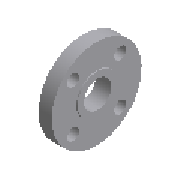
# Autodesk Inventor part: DIN EN 1092-2 Hubbed Slip-On Flange for Welding Type 12 - PN 63 Ductile Iron DN80
Saved by Autodesk Inventor 2024.2 (Build 282272000, 272)
## iProperties
Created: 2023-01-19
Part Number: DIN EN 1092-2 Hubbed Slip-On Flange for Welding Type 12 - PN 63 Ductile Iron DN80
Material: Iron, Ductile
Description: Flange
Document SubType Name: Modeling
Standard: DIN EN 1092-2
Designer: admin
Standards Organization: DIN
Language: en-US
Size Designation: DN80
Categories: <MemberInstance><Categories><Category DisplayName="Tube &amp; Pipe" InternalName="4347fa0f-2144-441d-94cd-e3e15c92b736" Mnemonic="TUBEANDPIPE"><CategoryParameter DisplayName="Number of Connections" InternalName="04e9c83a-9e20-4a98-a7e1-e8abe87a2846" Mnemonic="NUM_CONNECTIONS"/><CategoryParameter DisplayName="Angles" InternalName="0e0e4fa4-3bd3-4656-a22e-4e07c8c476f8" Mnemonic="ANGLES"><CategoryParameter DisplayName="Angle" InternalName="9188ad83-1b16-48b4-8b0a-76ce729dafa7" Mnemonic="ANGLE"/></CategoryParameter><CategoryParameter DisplayName="SKey" InternalName="3da84699-049a-4bc2-a65a-6696b77c242f" Mnemonic="SKEY"/><CategoryParameter DisplayName="ISOGEN Description" InternalName="7aa3ba45-b821-4467-8584-f9e6f15f2a7d" Mnemonic="ISOGENDESC"/><CategoryParameter DisplayName="ITEM-CODE" InternalName="99cc3b15-24d9-4d38-aac7-792cfbc57acf" Mnemonic="ITEMCODE"/><CategoryParameter DisplayName="NameOfComponent" InternalName="9c74ad13-48a1-45fe-b0f7-5447561f444a" Mnemonic="NAMEOFCOMPONENT"/><CategoryParameter DisplayName="InLineGroups" InternalName="d60be647-bc43-4c18-a13f-9fe4115f8e64" Mnemonic="INLINEGROUPS"/><Category DisplayName="Fittings" InternalName="ed6b26c4-72b8-4f31-9b63-f85ae8f932e4" Mnemonic="FITTINGS"><CategoryParameter DisplayName="Connections" InternalName="dbd721e8-e885-4eea-9011-b5acfd9f61de" Mnemonic="FIT_CONNECTIONS"><CategoryParameter DisplayName="Min Mating Pipe Size" InternalName="11f51b32-3e37-4310-abf7-f1318a1fd129" Mnemonic="MNMPS"/><CategoryParameter DisplayName="MaxEngagement" InternalName="34fdf028-8797-436e-ba07-ca3dee15bd9b" Mnemonic="MAXENGAGEMENT"/><CategoryParameter DisplayName="NominalSize" InternalName="3f94edc7-e459-48db-8f02-8eebf8cffccd" Mnemonic="NS"/><CategoryParameter DisplayName="DisplayName" InternalName="50f521dd-e050-43f7-9895-6b30ea7ed42e" Mnemonic="DISPLAYNAME"/><CategoryParameter DisplayName="Cut Mating Pipe" InternalName="53a63a6e-53d8-4ca9-8880-037731d1cceb" Mnemonic="CMP"/><CategoryParameter DisplayName="Gender Neutral" InternalName="628bd5f1-acad-44e2-9d91-af996ab74fc2" Mnemonic="NEUTRAL"/><CategoryParameter DisplayName="MinEngagement [% of MaxEngagement]" InternalName="7ec1bde5-73f0-45b1-98d8-365a6c67f8ad" Mnemonic="MINENGAGEMENT"/><CategoryParameter DisplayName="Fixed" InternalName="9142902a-6a8a-446d-9eb8-4b7ce7d245ef" Mnemonic="FIXED"/><CategoryParameter DisplayName="Female" InternalName="b366bcb5-a500-4bad-84bb-22f956216d69" Mnemonic="FEMALE"/><CategoryParameter DisplayName="FlipDirection" InternalName="d55dedc0-f14a-4283-86b4-a4eeb253c8aa" Mnemonic="FLIPDIRECTION"/><CategoryParameter DisplayName="ScheduleNumber" InternalName="d6161c62-eb59-4495-a086-874847c10866" Mnemonic="SN"/><CategoryParameter DisplayName="EndTreatment" InternalName="d7f11516-3374-45ca-b1c7-4b2d63244ae2" Mnemonic="ENDTREATMENT"/><CategoryParameter DisplayName="Max Mating Pipe Size" InternalName="e73ef66b-c04b-45ac-9b32-f712653e25ee" Mnemonic="MXMPS"/></CategoryParameter><CategoryParameter DisplayName="Connections" InternalName="dbd721e8-e885-4eea-9011-b5acfd9f61de" Mnemonic="FIT_CONNECTIONS"><CategoryParameter DisplayName="Min Mating Pipe Size" InternalName="11f51b32-3e37-4310-abf7-f1318a1fd129" Mnemonic="MNMPS"/><CategoryParameter DisplayName="MaxEngagement" InternalName="34fdf028-8797-436e-ba07-ca3dee15bd9b" Mnemonic="MAXENGAGEMENT"/><CategoryParameter DisplayName="NominalSize" InternalName="3f94edc7-e459-48db-8f02-8eebf8cffccd" Mnemonic="NS"/><CategoryParameter DisplayName="DisplayName" InternalName="50f521dd-e050-43f7-9895-6b30ea7ed42e" Mnemonic="DISPLAYNAME"/><CategoryParameter DisplayName="Cut Mating Pipe" InternalName="53a63a6e-53d8-4ca9-8880-037731d1cceb" Mnemonic="CMP"/><CategoryParameter DisplayName="Gender Neutral" InternalName="628bd5f1-acad-44e2-9d91-af996ab74fc2" Mnemonic="NEUTRAL"/><CategoryParameter DisplayName="MinEngagement [% of MaxEngagement]" InternalName="7ec1bde5-73f0-45b1-98d8-365a6c67f8ad" Mnemonic="MINENGAGEMENT"/><CategoryParameter DisplayName="Fixed" InternalName="9142902a-6a8a-446d-9eb8-4b7ce7d245ef" Mnemonic="FIXED"/><CategoryParameter DisplayName="Female" InternalName="b366bcb5-a500-4bad-84bb-22f956216d69" Mnemonic="FEMALE"/><CategoryParameter DisplayName="FlipDirection" InternalName="d55dedc0-f14a-4283-86b4-a4eeb253c8aa" Mnemonic="FLIPDIRECTION"/><CategoryParameter DisplayName="ScheduleNumber" InternalName="d6161c62-eb59-4495-a086-874847c10866" Mnemonic="SN"/><CategoryParameter DisplayName="EndTreatment" InternalName="d7f11516-3374-45ca-b1c7-4b2d63244ae2" Mnemonic="ENDTREATMENT"/><CategoryParameter DisplayName="Max Mating Pipe Size" InternalName="e73ef66b-c04b-45ac-9b32-f712653e25ee" Mnemonic="MXMPS"/></CategoryParameter><Category DisplayName="Flanges" InternalName="77d2c0aa-3125-426d-b447-5c3546f42b82" Mnemonic="Flange"/></Category></Category><Category DisplayName="DataType" InternalName="23b78d0f-2648-40c6-8793-ca6db495c9e8" Mnemonic="DATATYPE"><CategoryParameter DisplayName="DisplayName" InternalName="05415f3d-3907-474b-a020-eb9d644f4cf3" Mnemonic="DISPLAYNAME"/><CategoryParameter DisplayName="Standard" InternalName="0c0a119c-1e12-4c84-803f-101930972f5e" Mnemonic="STANDARD"/><CategoryParameter DisplayName="Description" InternalName="13903e3d-64b1-4950-80da-f627842ea37f" Mnemonic="DESCRIPTION"/><CategoryParameter DisplayName="Designation" InternalName="2675968c-4ce5-49e0-a4f5-552d29089031" Mnemonic="DESIGNATION"/><CategoryParameter DisplayName="Default Row" InternalName="2af9ec52-faaa-4026-b378-f9fa4afca842" Mnemonic="DEFAULTROW"/><CategoryParameter DisplayName="Folder Name" InternalName="3f06958e-8713-4116-9be7-ed6184ecc97b" Mnemonic="FOLDERNAME"/><CategoryParameter DisplayName="Revision Guid" InternalName="45a75005-10b1-4dfc-8d6d-dfe629f0b93c" Mnemonic="REVISIONGUID"/><CategoryParameter DisplayName="FileName" InternalName="8b46a4cc-9585-4fed-90c3-899f57e09a73" Mnemonic="FILENAME"/><CategoryParameter DisplayName="StdsOrg" InternalName="8f5914e1-4693-403f-8ab5-d37768198c9d" Mnemonic="STDSORG"/><CategoryParameter DisplayName="Family Version" InternalName="914462f6-6e19-4b14-ba84-155b9680b1d0" Mnemonic="FAMILYREVISION"/><CategoryParameter DisplayName="Standard Revision" InternalName="91d5a463-65c2-4fde-b823-3b7fea5e8e17" Mnemonic="STANDARDREVISION"/><CategoryParameter DisplayName="Member Revision" InternalName="a65d44b9-392f-4f4f-857b-e4b3d54996fe" Mnemonic="MEMBERREVISION"/><CategoryParameter DisplayName="ClipFormat" InternalName="bc51e27b-3422-4e78-93ef-cec197ddf230" Mnemonic="CLIPFORMAT"/><CategoryParameter DisplayName="Manufacturer" InternalName="cd6c7a72-a28a-4e50-99a9-2c7f4e13e5ad" Mnemonic="MANUFACTURER"/><CategoryParameter DisplayName="InternalName" InternalName="cf1d0246-76d9-4b4a-8305-fa0409afb5c1" Mnemonic="INTERNALNAME"/><CategoryParameter DisplayName="IsMetric" InternalName="e2385c5b-1ea4-4823-96a8-8de651266ec3" Mnemonic="ISMETRIC"/><Category DisplayName="Part" InternalName="c0e0b642-3bcb-4cc8-9e80-f96d35c4afa4" Mnemonic="PART"><CategoryParameter DisplayName="Part Number" InternalName="016b6077-bfbe-49bd-92c9-d8d59c39c941" Mnemonic="PARTNUMBER"/><CategoryParameter DisplayName="Stock Number" InternalName="4dba7c1c-e26c-444e-836c-b08b433409a8" Mnemonic="STOCKNUMBER"/><CategoryParameter DisplayName="Material Key" InternalName="5c9a8adb-dd2b-4535-b97f-0a94a95fe41f" Mnemonic="MATERIALKEY"/><CategoryParameter DisplayName="Material" InternalName="818a152a-d3c3-49ca-80ee-df7d91421b8e" Mnemonic="MATERIAL"/></Category></Category><Category DisplayName="LegacyMap" InternalName="dfeab48a-acc2-4514-a11c-1b8dc28c3d5f" Mnemonic="LEGACYMAP"><CategoryParameter DisplayName="CatalogID" InternalName="0da51c36-8fd3-4028-86cc-0c9c9e96136a" Mnemonic="CATALOGID"/><CategoryParameter DisplayName="FamilyID" InternalName="1c0b589c-8bbe-4e1e-80cf-07c0de42ac2a" Mnemonic="FAMILYID"/><CategoryParameter DisplayName="MemberID" InternalName="a368ea03-db8a-4d6e-962b-2aa46306b8f5" Mnemonic="MEMBERID"/></Category></Categories><FamilyTemplate Id="DIN EN 1092-2 Hubbed Slip-On Flange for Welding Type 12 - PN 63 Ductile Iron"><FamilyTemplateParameters><FamilyTemplateParameter ObjectType="kUserParameterObject" ValueType="xs:integer" Id="1" ObjectReferenceKey="NU"/><FamilyTemplateParameter ObjectType="kUserParameterObject" ValueType="xs:double" Id="2" ObjectReferenceKey="D"/><FamilyTemplateParameter ObjectType="kUserParameterObject" ValueType="xs:double" Id="3" ObjectReferenceKey="K1"/><FamilyTemplateParameter ObjectType="kUserParameterObject" ValueType="xs:double" Id="4" ObjectReferenceKey="L"/><FamilyTemplateParameter ObjectType="kUserParameterObject" ValueType="xs:double" Id="5" ObjectReferenceKey="C1"/><FamilyTemplateParameter ObjectType="kUserParameterObject" ValueType="xs:double" Id="6" ObjectReferenceKey="D1"/><FamilyTemplateParameter ObjectType="kUserParameterObject" ValueType="xs:double" Id="7" ObjectReferenceKey="F1"/><FamilyTemplateParameter ObjectType="kUserParameterObject" ValueType="xs:double" Id="8" ObjectReferenceKey="H2"/><FamilyTemplateParameter ObjectType="kUserParameterObject" ValueType="xs:double" Id="9" ObjectReferenceKey="N3"/><FamilyTemplateParameter ObjectType="kUserParameterObject" ValueType="xs:double" Id="10" ObjectReferenceKey="ID"/><FamilyTemplateParameter ObjectType="kUserParameterObject" ValueType="xs:double" Id="11" ObjectReferenceKey="t"/><FamilyTemplateParameter ObjectType="kUserParameterObject" ValueType="xs:string" Id="120" ObjectReferenceKey="Size_Designation"/><FamilyTemplateParameter ObjectType="kPropertyObject" ValueType="xs:string" Id="100" ObjectReferenceKey="{32853F0F-3444-11d1-9E93-0060B03C1CA6}" SubObjectId="52"/><FamilyTemplateParameter ObjectType="kPropertyObject" ValueType="xs:string" Id="105" ObjectReferenceKey="{32853F0F-3444-11d1-9E93-0060B03C1CA6}" SubObjectId="5"/><FamilyTemplateParameter ObjectType="kPartComponentDefinitionObject" ValueType="xs:string" Id="110" SubObjectId="Material"/></FamilyTemplateParameters></FamilyTemplate><CategoryParameterMap><ParamToTemplateMap><ParamToTemplate CategoryParameter="//CategoryParameter[@InternalName='d60be647-bc43-4c18-a13f-9fe4115f8e64']" ConstantValue="1"/><ParamToTemplate CategoryParameter="//CategoryParameter[@InternalName='04e9c83a-9e20-4a98-a7e1-e8abe87a2846']" ConstantValue="2"/><ParamToTemplate CategoryParameter="//CategoryParameter[@InternalName='0e0e4fa4-3bd3-4656-a22e-4e07c8c476f8']" ConstantValue=""/><ParamToTemplate CategoryParameter="//CategoryParameter[@InternalName='0e0e4fa4-3bd3-4656-a22e-4e07c8c476f8'][1]/CategoryParameter[@InternalName='9188ad83-1b16-48b4-8b0a-76ce729dafa7']" ConstantValue="3.14159265358979"/><ParamToTemplate CategoryParameter="//CategoryParameter[@InternalName='9c74ad13-48a1-45fe-b0f7-5447561f444a']" ConstantValue="FLANGE"/><ParamToTemplate CategoryParameter="//CategoryParameter[@InternalName='3da84699-049a-4bc2-a65a-6696b77c242f']" ConstantValue="FLSO"/><ParamToTemplate CategoryParameter="//CategoryParameter[@InternalName='dbd721e8-e885-4eea-9011-b5acfd9f61de'][1]/CategoryParameter[@InternalName='d55dedc0-f14a-4283-86b4-a4eeb253c8aa']" ConstantValue="true"/><ParamToTemplate CategoryParameter="//CategoryParameter[@InternalName='dbd721e8-e885-4eea-9011-b5acfd9f61de'][1]/CategoryParameter[@InternalName='50f521dd-e050-43f7-9895-6b30ea7ed42e']" ConstantValue="Connection1"/><ParamToTemplate CategoryParameter="//CategoryParameter[@InternalName='dbd721e8-e885-4eea-9011-b5acfd9f61de'][1]/CategoryParameter[@InternalName='b366bcb5-a500-4bad-84bb-22f956216d69']" ConstantValue="true"/><ParamToTemplate CategoryParameter="//CategoryParameter[@InternalName='dbd721e8-e885-4eea-9011-b5acfd9f61de'][1]/CategoryParameter[@InternalName='d7f11516-3374-45ca-b1c7-4b2d63244ae2']" ConstantValue="Flanged"/><ParamToTemplate CategoryParameter="//CategoryParameter[@InternalName='dbd721e8-e885-4eea-9011-b5acfd9f61de'][1]/CategoryParameter[@InternalName='9142902a-6a8a-446d-9eb8-4b7ce7d245ef']" ConstantValue="true"/><ParamToTemplate CategoryParameter="//CategoryParameter[@InternalName='dbd721e8-e885-4eea-9011-b5acfd9f61de'][1]/CategoryParameter[@InternalName='34fdf028-8797-436e-ba07-ca3dee15bd9b']" ConstantValue="0"/><ParamToTemplate CategoryParameter="//CategoryParameter[@InternalName='dbd721e8-e885-4eea-9011-b5acfd9f61de'][1]/CategoryParameter[@InternalName='7ec1bde5-73f0-45b1-98d8-365a6c67f8ad']" ConstantValue="0"/><ParamToTemplate CategoryParameter="//CategoryParameter[@InternalName='dbd721e8-e885-4eea-9011-b5acfd9f61de'][2]/CategoryParameter[@InternalName='d55dedc0-f14a-4283-86b4-a4eeb253c8aa']" ConstantValue="false"/><ParamToTemplate CategoryParameter="//CategoryParameter[@InternalName='dbd721e8-e885-4eea-9011-b5acfd9f61de'][2]/CategoryParameter[@InternalName='50f521dd-e050-43f7-9895-6b30ea7ed42e']" ConstantValue="Connection2"/><ParamToTemplate CategoryParameter="//CategoryParameter[@InternalName='dbd721e8-e885-4eea-9011-b5acfd9f61de'][2]/CategoryParameter[@InternalName='b366bcb5-a500-4bad-84bb-22f956216d69']" ConstantValue="true"/><ParamToTemplate CategoryParameter="//CategoryParameter[@InternalName='dbd721e8-e885-4eea-9011-b5acfd9f61de'][2]/CategoryParameter[@InternalName='d7f11516-3374-45ca-b1c7-4b2d63244ae2']" ConstantValue="Slip-on Welded"/><ParamToTemplate CategoryParameter="//CategoryParameter[@InternalName='dbd721e8-e885-4eea-9011-b5acfd9f61de'][2]/CategoryParameter[@InternalName='9142902a-6a8a-446d-9eb8-4b7ce7d245ef']" ConstantValue="false"/><ParamToTemplate CategoryParameter="//CategoryParameter[@InternalName='dbd721e8-e885-4eea-9011-b5acfd9f61de'][2]/CategoryParameter[@InternalName='34fdf028-8797-436e-ba07-ca3dee15bd9b']" ConstantValue="0"/><ParamToTemplate CategoryParameter="//CategoryParameter[@InternalName='dbd721e8-e885-4eea-9011-b5acfd9f61de'][2]/CategoryParameter[@InternalName='7ec1bde5-73f0-45b1-98d8-365a6c67f8ad']" ConstantValue="20"/><ParamToTemplate CategoryParameter="//CategoryParameter[@InternalName='dbd721e8-e885-4eea-9011-b5acfd9f61de'][1]/CategoryParameter[@InternalName='628bd5f1-acad-44e2-9d91-af996ab74fc2']" ConstantValue="true"/><ParamToTemplate CategoryParameter="//CategoryParameter[@InternalName='05415f3d-3907-474b-a020-eb9d644f4cf3']" ConstantValue="DIN EN 1092-2 Hubbed Slip-On Flange for Welding Type 12 - PN 63 Ductile Iron"/><ParamToTemplate CategoryParameter="//CategoryParameter[@InternalName='cf1d0246-76d9-4b4a-8305-fa0409afb5c1']" ConstantValue="134f9492-4b9a-4d81-9c99-863626225704"/><ParamToTemplate CategoryParameter="//CategoryParameter[@InternalName='3f06958e-8713-4116-9be7-ed6184ecc97b']" ConstantValue="DIN EN 1092-2 12 - PN 63"/><ParamToTemplate CategoryParameter="//CategoryParameter[@InternalName='914462f6-6e19-4b14-ba84-155b9680b1d0']" ConstantValue="10"/><ParamToTemplate CategoryParameter="//CategoryParameter[@InternalName='13903e3d-64b1-4950-80da-f627842ea37f']" ConstantValue="Flange"/><ParamToTemplate CategoryParameter="//CategoryParameter[@InternalName='8f5914e1-4693-403f-8ab5-d37768198c9d']" ConstantValue="DIN"/><ParamToTemplate CategoryParameter="//CategoryParameter[@InternalName='0c0a119c-1e12-4c84-803f-101930972f5e']" ConstantValue="DIN EN 1092-2"/><ParamToTemplate CategoryParameter="//CategoryParameter[@InternalName='cd6c7a72-a28a-4e50-99a9-2c7f4e13e5ad']" TemplateParameter="104"/><ParamToTemplate CategoryParameter="//CategoryParameter[@InternalName='91d5a463-65c2-4fde-b823-3b7fea5e8e17']" TemplateParameter="103"/><ParamToTemplate CategoryParameter="//CategoryParameter[@InternalName='bc51e27b-3422-4e78-93ef-cec197ddf230']" ConstantValue="CF_INVENTOR.STDPARTS"/><ParamToTemplate CategoryParameter="//CategoryParameter[@InternalName='e2385c5b-1ea4-4823-96a8-8de651266ec3']" ConstantValue="true"/><ParamToTemplate CategoryParameter="//CategoryParameter[@InternalName='45a75005-10b1-4dfc-8d6d-dfe629f0b93c']" ConstantValue="40f8a042-b52d-47fe-82f4-b6fd9baced96"/><ParamToTemplate CategoryParameter="//CategoryParameter[@InternalName='2af9ec52-faaa-4026-b378-f9fa4afca842']" ConstantValue="1"/><ParamToTemplate CategoryParameter="//CategoryParameter[@InternalName='0da51c36-8fd3-4028-86cc-0c9c9e96136a']" ConstantValue="4126CA90-F456-496D-BC37-DD4E9B6C39DC"/><ParamToTemplate CategoryParameter="//CategoryParameter[@InternalName='1c0b589c-8bbe-4e1e-80cf-07c0de42ac2a']" ConstantValue="134f9492-4b9a-4d81-9c99-863626225704"/><ParamToTemplate CategoryParameter="//CategoryParameter[@InternalName='99cc3b15-24d9-4d38-aac7-792cfbc57acf']" ConstantValue=""/><ParamToTemplate CategoryParameter="//CategoryParameter[@InternalName='7aa3ba45-b821-4467-8584-f9e6f15f2a7d']" ConstantValue=""/><ParamToTemplate CategoryParameter="//CategoryParameter[@InternalName='dbd721e8-e885-4eea-9011-b5acfd9f61de'][1]/CategoryParameter[@InternalName='3f94edc7-e459-48db-8f02-8eebf8cffccd']" ConstantValue="M80"/><ParamToTemplate CategoryParameter="//CategoryParameter[@InternalName='dbd721e8-e885-4eea-9011-b5acfd9f61de'][2]/CategoryParameter[@InternalName='3f94edc7-e459-48db-8f02-8eebf8cffccd']" ConstantValue="M80"/><ParamToTemplate CategoryParameter="//CategoryParameter[@InternalName='8b46a4cc-9585-4fed-90c3-899f57e09a73']" ConstantValue="DIN EN 1092-2 Hubbed Slip-On Flange for Welding Type 12 - PN 63 Ductile Iron DN80"/><ParamToTemplate CategoryParameter="//CategoryParameter[@InternalName='a65d44b9-392f-4f4f-857b-e4b3d54996fe']" ConstantValue="2A3BDD21-11B0-47DD-9341-421F42603EF8"/><ParamToTemplate CategoryParameter="//CategoryParameter[@InternalName='a368ea03-db8a-4d6e-962b-2aa46306b8f5']" ConstantValue="E22A34FC-127D-40B1-BA5F-93BBAD1B1EE2"/><ParamToTemplate CategoryParameter="//CategoryParameter[@InternalName='2675968c-4ce5-49e0-a4f5-552d29089031']" TemplateParameter="100"/><ParamToTemplate CategoryParameter="//CategoryParameter[@InternalName='818a152a-d3c3-49ca-80ee-df7d91421b8e']" TemplateParameter="110"/><ParamToTemplate CategoryParameter="//CategoryParameter[@InternalName='016b6077-bfbe-49bd-92c9-d8d59c39c941']" TemplateParameter="105"/></ParamToTemplateMap></CategoryParameterMap></MemberInstance>
Density: 7.15 g/cm^3
Appearance: Iron Gray
NAME: PIPING: DIN EN 1092-2 Hubbed Slip-On Flange for Welding Type 12 - PN 63 Ductile Iron
DATA: <meta><inlinegroups number="1" deflen="3"></inlinegroups><connections number="2"></connections><angles><a>3.14159265358979</a></angles></meta>
IsCustomPart: 0
Author: admin
Autodesk Inventor part; units mm, degrees
ref_plane "YZ Plane" through (0, 0, 0) normal (1, 0, 0) x (0, 1, 0)
ref_plane "XZ Plane" through (0, 0, 0) normal (0, 1, 0) x (-1, 0, 0)
ref_plane "XY Plane" through (0, 0, 0) normal (0, 0, 1) x (1, 0, 0)
sketch "Sketch1" plane through (0, 0, 0) normal (0, 0, 1) x (1, 0, 0)
  line L0 (0, 0) -> (48, 0) construction
  line L1 (0, 46) -> (0, 66)
  line L2 (0, 66) -> (3, 66)
  line L3 (3, 107.5) -> (31, 107.5)
  line L4 (0, 46) -> (0, 0) construction
  line L5 (3, 107.5) -> (3, 66)
  line L6 (31, 107.5) -> (31, 61)
  line L7 (0, 46) -> (48, 46)
  line L8 (48, 46) -> (48, 0) construction
  line L9 (48, 59.5127) -> (31, 61)
  line L10 (48, 59.5127) -> (48, 46)
  dimension "d0" = 132
  dimension "d1" = 215
  dimension "d2" = 31
  dimension "d3" = 3
  dimension "d8" = 92
  dimension "d9" = 122
  dimension "d10" = 48
  dimension "d12" = 5
  constraints: 22 end point, 3 parallel, 3 perpendicular, 1 collinear, 1 horizontal
  measures "d0" diameter of L2 L0
  measures "d1" diameter of L3 L0
  measures "d2" distance between parallel lines of L1 L6
  measures "d3" distance between parallel lines of L1 L5
  measures "d8" diameter of L7 L0
  measures "d9" diameter of L6.end L0
  measures "d10" distance between parallel lines of L1 L10
  measures "d12" angle of L7 L9
revolve "Revolution1" add sketch "Sketch1" angle 360 about axis through (0, 0, 0) along (1, 0, 0)
sketch "Sketch2" plane through (3, 0, 0) normal (-1, 0, 0) x (0, 0, 1)
  circle A0 centre (0, 0) radius 66 projected
  line L0 (0, 0) -> (0, 85) construction
  circle A1 centre (0, 0) radius 107.5 projected
  circle A2 centre (0, 0) radius 85 construction
  line L1 (0, 0) -> (32.5281, 78.5298) construction
  circle A3 centre (32.5281, 78.5298) radius 11.5
  dimension "d13" = 23
  dimension "d14" = 85
  dimension "d15" = 22.5
  constraints: 4 end point, 2 centre point, 2 coincident, 2 point on circle, 1 vertical
  measures "d13" diameter of A3
  measures "d14" distance of L1.start L1.end
  measures "d15" angle of L1 L0
extrude "Extrusion1" cut sketch "Sketch2" against normal blind 31 contours A3
pattern_circular "Circular Pattern1" count 8 over 360 about axis through (1.5, 0, 0) along (1, 0, 0) of "Extrusion1"
equation "\"d0\" = D1"
equation "\"d1\" = D"
equation "\"d2\" = C1"
equation "\"d3\" = F1"
equation "\"d8\" = ID + 2 * t"
equation "\"d9\" = N3"
equation "\"d10\" = H2"
equation "\"d13\" = L"
equation "\"d14\" = 0.5 * K1"
equation "\"d4\" = C1"
equation "\"C1\" = 31"
equation "\"D\" = 215"
equation "\"L\" = 23"
equation "\"N3\" = 122"
equation "\"D1\" = 132"
equation "\"H2\" = 48"
equation "\"F1\" = 3"
equation "\"t\" = 6"
equation "\"Size_Designation\" = 1.2345"
equation "\"ID\" = 80"
equation "\"K1\" = 170"
body "Solid1"
